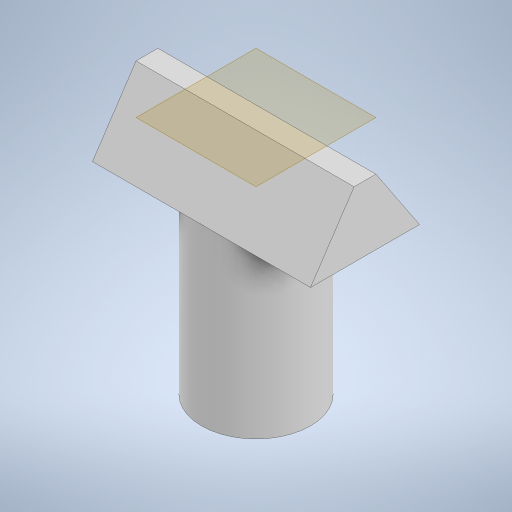
# Autodesk Inventor part: rotator_flat
Saved by Autodesk Inventor 2023.1 (Build 271208000, 208)
## iProperties
Created: 2022-10-07
Part Number: rotator_flat
Material: Generic
Document SubType Name: Modeling
Designer: swang
Density: 1 g/cm^3
Appearance: Default
Author: swang
Autodesk Inventor part; units mm, degrees
ref_plane "YZ Plane" through (0, 0, 0) normal (1, 0, 0) x (0, 1, 0)
ref_plane "XZ Plane" through (0, 0, 0) normal (0, 1, 0) x (-1, 0, 0)
ref_plane "XY Plane" through (0, 0, 0) normal (0, 0, 1) x (1, 0, 0)
sketch "Sketch1" plane through (0, 0, 0) normal (0, 1, 0) x (-1, 0, 0)
  circle A0 centre (0, 0) radius 25
  dimension "d0" = 50
  constraints: 1 centre point, 1 coincident
  measures "d0" diameter of A0
extrude "Extrusion1" add sketch "Sketch1" along normal blind 80
sketch "Sketch3" plane through (0, 80, 0) normal (0, 1, 0) x (1, 0, 0)
  line L0 (-50, -25) -> (50, -25)
  line L1 (50, -25) -> (50, 25)
  line L2 (50, 25) -> (-50, 25)
  line L3 (-50, 25) -> (-50, -25)
  line L4 (-50, -25) -> (50, 25) construction
  line L5 (50, -25) -> (-50, 25) construction
  point P0 (0, 0)
  dimension "d7" = 100
  dimension "d11" = 50
  constraints: 12 end point, 2 midpoint, 2 parallel, 1 horizontal, 1 perpendicular
  measures "d7" distance of L1.end L2.end
  measures "d11" distance of L0.end L1.end
ref_plane "Work Plane1" through (0, 110, 0) normal (0, 1, 0) x (1, 0, 0)
sketch "Sketch4" plane through (0, 110, 0) normal (0, 1, 0) x (1, 0, 0)
  line L0 (-50, -5) -> (50, -5)
  line L1 (50, -5) -> (50, 5)
  line L2 (50, 5) -> (-50, 5)
  line L3 (-50, 5) -> (-50, -5)
  line L4 (-50, -5) -> (50, 5) construction
  line L5 (50, -5) -> (-50, 5) construction
  point P0 (0, 0)
  dimension "d9" = 100
  dimension "d10" = 10
  constraints: 12 end point, 2 midpoint, 2 parallel, 1 horizontal, 1 perpendicular
  measures "d9" distance of L1.end L2.end
  measures "d10" distance of L0.end L1.end
loft "Loft1" add profiles "Sketch4", "Sketch3"
body "Solid1"
